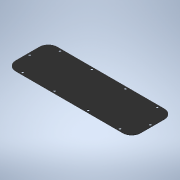
# Autodesk Inventor part: 1XX4_04_00_4(1)_P5
Saved by Autodesk Inventor 2021 (Build 250183000, 183)
## iProperties
Created: 2025-07-29
Part Number: 1XX4_04_00_4(1)_P5
Material: Generic
Catalog Web Link: www.cadenas.de
Description: AE 2.0 Flanschplatte-AE 2.0 Flanschplatte
Vendor: RITTAL
Document SubType Name: Modeling
Designer: psAdmin
Manufacturer: RITTAL
Mass: 97.9753 g
Surface Area: 1326.79 cm^2
Volume: 97.9753 cm^3
Density: 1 g/cm^3
Appearance: PSOLRGB-176-176-176
Category: PARTsolutions
Company: RITTAL
Title: 1XX4_04_00_4(1)_P5
Author: Cadenas PARTsolutions
Comments: AE 2.0 Flanschplatte
PSOL_IDENT_0: {$CADENAS_DATA/23d-libs/rittal/schaltschranksys/kompakt_schaltschr/parts_ae_2_0/flanschplatte_ae_2_0
PSOL_IDENT_1: .prj},203 {VTYP=3D},{NB=1XX4_04_00_4(1)_P5},{LINA=1XX4_04_00_4(1)_P5},{NN=AE 2.0 Flanschplatte},{DAT
PSOL_IDENT_2: E=28.04.2025 21:11:31},{GEOMDATE=11.04.2025 11:21:47},{VERSION=},{LINEID=110},{WBVAR=DETAIL},{WBNUME
PSOL_IDENT_3: RIC=DETAIL}  {NB=1XX4_04_00_4(1)_P5},{LINA=1XX4_04_00_4(1)_P5},{KT=DUMMY},{BEST=1XX4},{DETAIL=1},{BE
PSOL_IDENT_4: Z1=Neues Kompaktgehäuse},{BEZ2=Stahlblech},{BEZ3=eintürig},{B=360.000},{H=133.000},{T=4},{F=330},{G=
PSOL_IDENT_5: 355},{B1=431.000},{H1=0.000},{T1=210},{F1=330},{G1=355},{S=2.0},{ST=MIN},{GEW=-1.00000001504747e+30}
PSOL_IDENT_6: ,{VERS=4},{CNSECLASS51=27-18-01-02},{CNSECLASS70=27-18-01-01},{CNSECLASS80=27-18-01-01},{CNSETIM40=E
PSOL_IDENT_7: C000261}
NB: 1XX4_04_00_4(1)_P5
NN: AE 2.0 Flanschplatte
NT: AE 2.0 Flanschplatte
NBSYN: $BEST._04_00_$VERS.($DETAIL.)_P5
LINA: 1XX4_04_00_4(1)_P5
CATALOG: Rittal
BEST: 1XX4
DETAIL: hoch
BEZ1: Neues Kompaktgehäuse
BEZ2: Stahlblech
BEZ3: eintürig
B: 360
H: 133
T: 4
F: 330
G: 355
B1: 431
H1: 0
T1: 210
F1: 330
G1: 355
S: 2
ST: 0
GEW: -1.00000001504747e+30
VERS: 4
CNSECLASS70: 27-18-01-01
CNSECLASS80: 27-18-01-01
SUPPLIER: RITTAL
ARTICLENO: 1XX4_04_00_4(1)_P5
BOMINFO: 1XX4_04_00_4(1)_P5
CREATOR: CADENAS GmbH
Autodesk Inventor part; units mm, degrees
sketch "Sketch_4" plane through (0, 0, 0) normal (0, 1, 0) x (1, 0, 0)
  arc A0 (-223.5, -42.5) -> (-191.5, -74.5) centre (-191.5, -42.5) ccw
  line L0 (-191.5, -74.5) -> (191.5, -74.5)
  arc A1 (191.5, -74.5) -> (223.5, -42.5) centre (191.5, -42.5) ccw
  line L1 (223.5, -42.5) -> (223.5, 42.5)
  arc A2 (223.5, 42.5) -> (191.5, 74.5) centre (191.5, 42.5) ccw
  line L2 (191.5, 74.5) -> (-191.5, 74.5)
  arc A3 (-191.5, 74.5) -> (-223.5, 42.5) centre (-191.5, 42.5) ccw
  line L3 (-223.5, 42.5) -> (-223.5, -42.5)
  circle A4 centre (215.5, 0) radius 3.6
  circle A5 centre (174, -66.5) radius 3.6
  circle A6 centre (174, 66.5) radius 3.6
  circle A7 centre (60, -66.5) radius 3.6
  circle A8 centre (60, 66.5) radius 3.6
  circle A9 centre (-60, -66.5) radius 3.6
  circle A10 centre (-60, 66.5) radius 3.6
  circle A11 centre (-174, -66.5) radius 3.6
  circle A12 centre (-174, 66.5) radius 3.6
  circle A13 centre (-215.5, 0) radius 3.6
  constraints: 14 centre point, 8 end point, 8 point on circle
extrude "Extrusion1" add sketch "Sketch_4" along normal blind 1.5
ref_plane "FP_XY" through (0, 0, 0) normal (0, -1, 0) x (1, 0, 0)
ref_plane "FP_YZ" through (0, 0, 0) normal (1, 0, 0) x (0, 0, 1)
ref_plane "FP_ZX" through (0, 0, 0) normal (0, 0, 1) x (0, -1, 0)
ref_plane "to_Bolt_1_XY" through (-215.5, 0, 0) normal (0, 1, 0) x (1, 0, 0)
ref_plane "to_Bolt_1_YZ" through (-215.5, 0, 0) normal (1, 0, 0) x (0, 0, -1)
ref_plane "to_Bolt_1_ZX" through (-215.5, 0, 0) normal (0, 0, -1) x (0, 1, 0)
ref_plane "to_Bolt_1_1_XY" through (-174, 0, -66.5) normal (0, 1, 0) x (1, 0, 0)
ref_plane "to_Bolt_1_1_YZ" through (-174, 0, -66.5) normal (1, 0, 0) x (0, 0, -1)
ref_plane "to_Bolt_1_1_ZX" through (-174, 0, -66.5) normal (0, 0, -1) x (0, 1, 0)
ref_plane "to_Bolt_1_2_XY" through (-60, 0, -66.5) normal (0, 1, 0) x (1, 0, 0)
ref_plane "to_Bolt_1_2_YZ" through (-60, 0, -66.5) normal (1, 0, 0) x (0, 0, -1)
ref_plane "to_Bolt_1_2_ZX" through (-60, 0, -66.5) normal (0, 0, -1) x (0, 1, 0)
ref_plane "to_Bolt_1_3_XY" through (60, 0, -66.5) normal (0, 1, 0) x (1, 0, 0)
ref_plane "to_Bolt_1_3_YZ" through (60, 0, -66.5) normal (1, 0, 0) x (0, 0, -1)
ref_plane "to_Bolt_1_3_ZX" through (60, 0, -66.5) normal (0, 0, -1) x (0, 1, 0)
ref_plane "to_Bolt_1_4_XY" through (174, 0, -66.5) normal (0, 1, 0) x (1, 0, 0)
ref_plane "to_Bolt_1_4_YZ" through (174, 0, -66.5) normal (1, 0, 0) x (0, 0, -1)
ref_plane "to_Bolt_1_4_ZX" through (174, 0, -66.5) normal (0, 0, -1) x (0, 1, 0)
ref_plane "to_Bolt_1_5_XY" through (-174, 0, 66.5) normal (0, 1, 0) x (1, 0, 0)
ref_plane "to_Bolt_1_5_YZ" through (-174, 0, 66.5) normal (1, 0, 0) x (0, 0, -1)
ref_plane "to_Bolt_1_5_ZX" through (-174, 0, 66.5) normal (0, 0, -1) x (0, 1, 0)
ref_plane "to_Bolt_1_6_XY" through (-60, 0, 66.5) normal (0, 1, 0) x (1, 0, 0)
ref_plane "to_Bolt_1_6_YZ" through (-60, 0, 66.5) normal (1, 0, 0) x (0, 0, -1)
ref_plane "to_Bolt_1_6_ZX" through (-60, 0, 66.5) normal (0, 0, -1) x (0, 1, 0)
ref_plane "to_Bolt_1_7_XY" through (60, 0, 66.5) normal (0, 1, 0) x (1, 0, 0)
ref_plane "to_Bolt_1_7_YZ" through (60, 0, 66.5) normal (1, 0, 0) x (0, 0, -1)
ref_plane "to_Bolt_1_7_ZX" through (60, 0, 66.5) normal (0, 0, -1) x (0, 1, 0)
ref_plane "to_Bolt_1_8_XY" through (174, 0, 66.5) normal (0, 1, 0) x (1, 0, 0)
ref_plane "to_Bolt_1_8_YZ" through (174, 0, 66.5) normal (1, 0, 0) x (0, 0, -1)
ref_plane "to_Bolt_1_8_ZX" through (174, 0, 66.5) normal (0, 0, -1) x (0, 1, 0)
ref_plane "to_Bolt_2_XY" through (215.5, 0, 0) normal (0, 1, 0) x (1, 0, 0)
ref_plane "to_Bolt_2_YZ" through (215.5, 0, 0) normal (1, 0, 0) x (0, 0, -1)
ref_plane "to_Bolt_2_ZX" through (215.5, 0, 0) normal (0, 0, -1) x (0, 1, 0)
body "Solid1"
